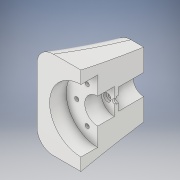
# Autodesk Inventor part: AA016
Saved by Autodesk Inventor 2017 SP1 (Build 210196100, 196)
## iProperties
Created: 2017-09-29
Part Number: AA016
Material: ABS Plastic
Document SubType Name: Modeling
Designer: Zach
Density: 1.06 g/cm^3
Appearance: CR White
Author: Zach
Autodesk Inventor part; units mm, degrees
ref_plane "YZ Plane" through (0, 0, 0) normal (1, 0, 0) x (0, 1, 0)
ref_plane "XZ Plane" through (0, 0, 0) normal (0, 1, 0) x (-1, 0, 0)
ref_plane "XY Plane" through (0, 0, 0) normal (0, 0, 1) x (1, 0, 0)
sketch "Sketch1" plane through (0, 0, 0) normal (0, 0, 1) x (1, 0, 0)
  line L0 (0, 0) -> (70, 0)
  line L1 (70, 0) -> (70, 77.5)
  line L2 (70, 77.5) -> (0, 77.5)
  line L3 (0, 77.5) -> (0, 0)
  dimension "d0" = 70
  dimension "d1" = 77.5
  constraints: 8 end point, 2 parallel, 1 horizontal, 1 perpendicular
  measures "d0" distance of L2.end L1.end
  measures "d1" distance of L1.end L0.end
extrude "Extrusion1" add sketch "Sketch1" along normal blind 75
sketch "Sketch3" plane through (0, 0, 75) normal (0, 0, 1) x (1, 0, 0)
  line L0 (0, 0) -> (70, 0) projected
  line L1 (70, 77.5) -> (0, 77.5) projected
  line L2 (70, 0) -> (35, 0)
  line L3 (35, 0) -> (35, 77.5)
  line L4 (35, 77.5) -> (70, 77.5)
  line L5 (70, 77.5) -> (70, 0)
  constraints: 8 end point, 2 parallel, 1 horizontal, 1 midpoint, 1 perpendicular
extrude "Extrusion3" cut sketch "Sketch3" against normal through all
sketch "Sketch4" plane through (0, 77.5, 75) normal (0, 1, 0) x (1, 0, 0)
  line L0 (0, 75) -> (0, 0) projected
  line L1 (0, 0) -> (-17.5, 0)
  line L2 (35, 75) -> (0, 75) projected
  arc A0 (-17.5, 0) -> (0, 75) centre (-1128.0394, 298.6675) ccw
  dimension "d8" = 17.5
  dimension "d9" = 1150
  constraints: 2 end point, 2 point on circle, 1 centre point, 1 horizontal
  measures "d8" distance of L0.end L1.end
  measures "d9" radius of A0
extrude "Extrusion4" add sketch "Sketch4" against normal blind 77.5
sketch "Sketch5" plane through (35, 0, 75) normal (1, 0, 0) x (0, 0, -1)
  line L0 (0, 77.5) -> (0, 91.25)
  line L1 (0, 0) -> (0, -13.75)
  line L2 (0, 0) -> (0, 77.5) projected
  line L3 (75, 77.5) -> (75, 0) projected
  arc A0 (0, 91.25) -> (75, 77.5) centre (244.7631, 1214.9008) ccw
  arc A1 (75, 0) -> (0, -13.75) centre (244.7631, -1137.4008) ccw
  line L4 (0, 77.5) -> (75, 77.5) projected
  line L5 (75, 0) -> (0, 0) projected
  dimension "d12" = 13.75
  dimension "d13" = 13.75
  dimension "d14" = 1150
  dimension "d15" = 1150
  constraints: 4 end point, 4 point on circle, 2 centre point, 2 vertical
  measures "d12" distance of L0.start L0.end
  measures "d13" distance of L1.start L1.end
  measures "d14" radius of A0
  measures "d15" radius of A1
extrude "Extrusion5" add sketch "Sketch5" against normal blind 55 contours L0 A0 L4 | L5 A1 L1
sketch "Sketch6" plane through (-20, 0, 0) normal (0, 1, 0) x (1, 0, 0)
  line L0 (20, 0) -> (0, 0) projected
  line L1 (0, -75) -> (0, 0) projected
  arc A0 (2.5, -75) -> (20, 0) centre (-1108.0394, 223.6675) ccw projected
  line L2 (2.5, -75) -> (0, -75) projected
extrude "Extrusion6" cut sketch "Sketch6" along normal through all both and the other way through all
fillet "Fillet3" radius 20 2 edges at (-8.1958, 83.8172, 37.9626) (-8.1958, -6.3172, 37.9626)
sketch "Sketch8" plane through (0, 0, 75) normal (0, 0, 1) x (1, 0, 0)
  line L0 (35, 91.25) -> (35, -13.75) projected
  line L1 (35, 77.5) -> (35, 0) projected
  circle A0 centre (35, 38.75) radius 37.5
  point P0 (0, 0)
  dimension "d23" = 75
  constraints: 1 centre point, 1 midpoint
  measures "d23" diameter of A0
extrude "Extrusion7" cut sketch "Sketch8" against normal blind 20
sketch "Sketch9" plane through (0, 0, 55) normal (0, 0, 1) x (1, 0, 0)
  line L0 (35, 76.25) -> (35, 1.25) projected
  circle A0 centre (35, 38.75) radius 15.5
  point P0 (0, 0)
  dimension "d26" = 31
  constraints: 1 centre point, 1 midpoint
  measures "d26" diameter of A0
extrude "Extrusion8" cut sketch "Sketch9" against normal blind 20
sketch "Sketch10" plane through (0, 0, 0) normal (0, 0, -1) x (-1, 0, 0)
  line L0 (-35, 77.5) -> (-35, 0) projected
  circle A0 centre (-35, 38.75) radius 12.5
  point P0 (0, 0)
  dimension "d29" = 25
  constraints: 1 centre point, 1 midpoint
  measures "d29" diameter of A0
extrude "Extrusion9" cut sketch "Sketch10" against normal blind 30
sketch "Sketch11" plane through (0, 0, 30) normal (0, 0, -1) x (-1, 0, 0)
  line L0 (-35, 26.25) -> (-35, 51.25) projected
  circle A0 centre (-35, 38.75) radius 2.5
  circle A1 centre (-26.5, 38.75) radius 2
  point P0 (0, 0)
  dimension "d32" = 5
  dimension "d33" = 4
  dimension "d34" = 8.5
  constraints: 3 midpoint, 2 centre point, 2 horizontal alignment
  measures "d32" diameter of A0
  measures "d33" diameter of A1
  measures "d34" distance of A0.centre A1.centre
extrude "Extrusion10" cut sketch "Sketch11" against normal through all
sketch "Sketch12" plane through (0, 0, 35) normal (0, 0, 1) x (1, 0, 0)
  circle A0 centre (26.5, 38.75) radius 2 projected
  circle A1 centre (26.5, 38.75) radius 4.5
  point P0 (0, 0)
  dimension "d37" = 9
  constraints: 1 centre point, 1 coincident
  measures "d37" diameter of A1
extrude "Extrusion11" cut sketch "Sketch12" against normal blind 3
sketch "Sketch14" plane through (0, 0, 30) normal (0, 0, -1) x (-1, 0, 0)
  arc A0 (-35, 36.25) -> (-35, 41.25) centre (-35, 38.75) ccw projected
  circle A1 centre (-35, 38.75) radius 4
  point P0 (0, 0)
  dimension "d40" = 8
  constraints: 1 centre point, 1 coincident
  measures "d40" diameter of A1
extrude "Extrusion12" cut sketch "Sketch14" against normal blind 3
sketch "Sketch15" plane through (0, 0, 55) normal (0, 0, 1) x (1, 0, 0)
  arc A0 (35, 41.25) -> (35, 36.25) centre (35, 38.75) ccw projected
  circle A1 centre (10, 38.75) radius 2.5
  circle A2 centre (22.5, 17.0994) radius 2.5
  circle A3 centre (47.5, 17.0994) radius 2.5
  circle A4 centre (60, 38.75) radius 2.5
  circle A5 centre (47.5, 60.4006) radius 2.5
  circle A6 centre (22.5, 60.4006) radius 2.5
  point P0 (0, 0)
  dimension "d43" = 5
  dimension "d44" = 25
  dimension "d47" = 360
  constraints: 6 centre point, 1 horizontal alignment, 13 other
  measures "d43" diameter of A1
  measures "d44" distance of A0.centre A1.centre
extrude "Extrusion13" cut sketch "Sketch15" against normal blind 25
body "Solid1"
